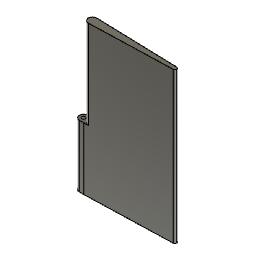
AletaAerodeslizador v1 (Autodesk Fusion 360 design; units mm, degrees)
Autodesk Fusion 360 part; units mm, degrees
sketch "Boceto1" plane through (0, 0, 0) normal (0, 0, 1) x (1, 0, 0)
  line L0 (0, 0) -> (0, 5)
  line L1 (0, 5) -> (0, 0)
  line L2 (0, 0) -> (0, -5)
  line L3 (0, 0) -> (100, 0)
  line L4 (100, 0) -> (100, -2)
  line L5 (100, 0) -> (100, 2)
  line L6 (0, 5) -> (100, 2)
  line L7 (100, -2) -> (0, -5)
  dimension "d1" = 100
  dimension "d2" = 2
  dimension "d3" = 2
  constraint coincident L0.start L1.end
  constraint vertical L0
  constraint parallel L0 L2
  constraint perpendicular L2 L3
  constraint perpendicular L3 L4
  constraint perpendicular L3 L5
  measures "d1" distance of L0.start L3.end
  measures "d2" distance of L3.end L4.end
  measures "d3" distance of L3.end L5.end
extrude "Extruir1" add sketch "Boceto1" along normal blind 170
sketch "Boceto2" plane through (0, 0, 0) normal (-1, 0, 0) x (0, -1, 0)
  line L0 (-5, 0) -> (5, 0)
  line L1 (5, 0) -> (5, 170)
  line L2 (5, 170) -> (-5, 170)
  line L3 (-5, 170) -> (-5, 0)
  line L4 (-5, 0) -> (5, 0)
  line L5 (5, 0) -> (5, 70)
  line L6 (5, 70) -> (-5, 70)
  line L7 (-5, 70) -> (-5, 0)
  dimension "d6" = 70
  constraint horizontal L4
  constraint vertical L5
  constraint horizontal L6
  constraint vertical L7
  constraint coincident L0.start L3.end
  measures "d6" distance of L0.start L6.end
extrude "Extruir2" add sketch "Boceto2" along normal blind 10 contours L0 L1 L3 L4 L5 L6 L7
sketch "Boceto3" plane through (0, 0, 70) normal (0, 0, 1) x (-1, 0, 0)
  line L0 (0, 5) -> (0, -5)
  line L1 (0, -5) -> (10, -5)
  line L2 (10, -5) -> (10, 5)
  line L3 (10, 5) -> (0, 5)
  line L4 (10, 0) -> (5, 0)
  circle A0 centre (5, 0) radius 2
  dimension "d9" = 4
  constraint midpoint L2 L4.start
  constraint perpendicular L0 L4
  constraint coincident L4.end A0.centre
  measures "d9" diameter of A0
extrude "Extruir3" cut sketch "Boceto3" against normal blind 70 contours A0
fillet "Empalme1" radius 5 2 edges at (-10, 5, 35) (-10, -5, 35)
fillet "Empalme2" radius 5 2 edges at (0, 5, 120) (0, -5, 120)
fillet "Empalme3" radius 2 2 edges at (100, -2, 85) (100, 2, 85)
